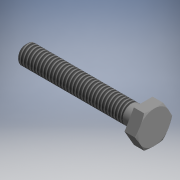
# Autodesk Inventor part: Hexagon bolt DIN 933 - M4x25
Saved by Autodesk Inventor 2017.3 (Build 213256000, 256)
## iProperties
Part Number: Hexagon bolt DIN 933 - M4x25
Material: Generic
Catalog Web Link: www.cadenas.de
Description: DIN 933-Hexagon bolt with thread to the head, product classes A and B, DIN 933 was replaced by ISO 24017
Vendor: FESTO
Document SubType Name: Modeling
Designer: partserver
Manufacturer: FESTO
Mass: 0.426226 g
Surface Area: 4.58956 cm^2
Volume: 0.426226 cm^3
Density: 1 g/cm^3
Appearance: PSOLRGB-175-175-175
Category: PARTsolutions
Company: FESTO
Title: Hexagon bolt DIN 933 - M4x25
Author: Cadenas PARTsolutions
Comments: Hexagon bolt with thread to the head, product classes A and B, DIN 933 was replaced by ISO 24017
PSOL_IDENT_0: {$CADENAS_DATA\23d-libs\festo\zyl_zubeh\din_933\din_933.prj},200 {VTYP=3D},{NB=Hexagon bolt DIN 933
PSOL_IDENT_1: - M4x25},{LINA=Hexagon bolt DIN 933 - M4x25},{NN=DIN 933},{DATE=06.11.2018 13:35:08},{GEOMDATE=06.11
PSOL_IDENT_2: .2018 13:35:02},{VERSION=v4},{LINEID=390},{WBVAR=},{WBNUMERIC=}  {NB=Sechskantschraube DIN 933 - M4x
PSOL_IDENT_3: 25},{LINA=Sechskantschraube DIN 933 - M4x25},{KT=X},{IDNR=},{NENN=M4x25},{D=4.000},{D3=3.141},{P=0.7
PSOL_IDENT_4: 00},{L=25.000},{S=7.000},{A=2.100},{C=0.400},{DA=4.700},{DW=6.030},{E=7.660},{K=2.800},{R=0.200}
NB: Hexagon bolt DIN 933 - M4x25
NN: DIN 933
NT: Hexagon bolt with thread to the head, product classes A and B, DIN 933 was replaced by ISO 24017
NBSYN: Hexagon bolt DIN 933 - $NENN.
LINA: Hexagon bolt DIN 933 - M4x25
CATALOG: Festo
ROWDESC: M4x25
D: 4
D3: 3.141
P: 0.7
L: 25
S: 7
A: 2.1
C: 0.4
DA: 4.7
DW: 6.03
E: 7.66
K: 2.8
R: 0.2
SUPPLIER: FESTO
ARTICLENO: Hexagon bolt DIN 933 - M4x25
BOMINFO: Hexagon bolt DIN 933 - M4x25
CREATOR: CADENAS GmbH
Autodesk Inventor part; units mm, degrees
ref_plane "YZ Plane" through (0, 0, 0) normal (1, 0, 0) x (0, 1, 0)
ref_plane "XZ Plane" through (0, 0, 0) normal (0, 1, 0) x (-1, 0, 0)
ref_plane "XY Plane" through (0, 0, 0) normal (0, 0, 1) x (1, 0, 0)
sketch "Skizze_1" plane through (0, 0, 0) normal (0, 0, 1) x (1, 0, 0)
  line L0 (25, 0) -> (-2.8, 0)
  line L1 (-2.8, 0) -> (-2.8, 3.5)
  line L2 (-2.8, 3.5) -> (-2.0357, 5.6)
  line L3 (-2.0357, 5.6) -> (-0.4, 5.6)
  line L4 (-0.4, 5.6) -> (-0.4, 3.015)
  line L5 (-0.4, 3.015) -> (0, 3.015)
  line L6 (0, 3.015) -> (0, 2.2)
  arc A0 (0, 2.2) -> (0.2, 2) centre (0.2, 2.2) ccw
  line L7 (0.2, 2) -> (24.5705, 2)
  line L8 (24.5705, 2) -> (25, 1.5705)
  line L9 (25, 1.5705) -> (25, 0)
  line L10 (25, 0) -> (-2.8, 0)
  constraints: 22 end point, 2 point on circle, 1 centre point
revolve "Revolution1" add sketch "Skizze_1" angle 360 about axis through (25, 0, 0) along (1, 0, 0)
thread "Thread1" size "M4x0.7" class "6g" standard "ISO Metric profile" length 22.4705
sketch "Skizze_2" plane through (0, 0, 0) normal (1, 0, 0) x (0, 0, -1)
  line L0 (-7, -7) -> (7, -7)
  line L1 (7, -7) -> (7, 7)
  line L2 (7, 7) -> (-7, 7)
  line L3 (-7, 7) -> (-7, -7)
  line L4 (-3.5, -2.0207) -> (0, -4.0415)
  line L5 (0, -4.0415) -> (3.5, -2.0207)
  line L6 (3.5, -2.0207) -> (3.5, 2.0207)
  line L7 (3.5, 2.0207) -> (0, 4.0415)
  line L8 (0, 4.0415) -> (-3.5, 2.0207)
  line L9 (-3.5, 2.0207) -> (-3.5, -2.0207)
  constraints: 20 end point
extrude "Extrusion1" cut sketch "Skizze_2" against normal blind 2.8
ref_plane "IP1_XY" through (0, 0, 0) normal (1, 0, 0) x (0, 0, -1)
ref_plane "IP1_YZ" through (0, 0, 0) normal (0, 0, -1) x (0, 1, 0)
ref_plane "IP1_ZX" through (0, 0, 0) normal (0, 1, 0) x (1, 0, 0)
ref_plane "IP2_XY" through (-2.8, 0, 0) normal (1, 0, 0) x (0, 0, -1)
ref_plane "IP2_YZ" through (-2.8, 0, 0) normal (0, 0, -1) x (0, 1, 0)
ref_plane "IP2_ZX" through (-2.8, 0, 0) normal (0, 1, 0) x (1, 0, 0)
ref_plane "IP3_XY" through (25, 0, 0) normal (1, 0, 0) x (0, 0, -1)
ref_plane "IP3_YZ" through (25, 0, 0) normal (0, 0, -1) x (0, 1, 0)
ref_plane "IP3_ZX" through (25, 0, 0) normal (0, 1, 0) x (1, 0, 0)
body "Solid1"
